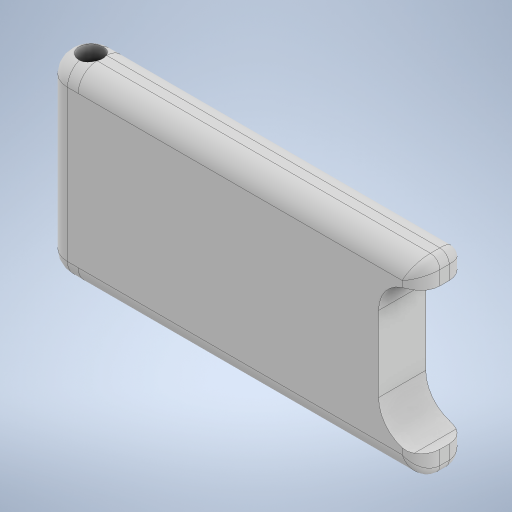
# Autodesk Inventor part: Brazo2_2
Saved by Autodesk Inventor 2024 (Build 280153000, 153)
## iProperties
Created: 2023-09-22
Part Number: Brazo2_2
Material: Genérico
Document SubType Name: Modeling
Designer: sergi
Density: 1 g/cm^3
Appearance: Valor por defecto
Author: sergi
Autodesk Inventor part; units mm, degrees
ref_plane "YZ Plane" through (0, 0, 0) normal (1, 0, 0) x (0, 1, 0)
ref_plane "XZ Plane" through (0, 0, 0) normal (0, 1, 0) x (-1, 0, 0)
ref_plane "XY Plane" through (0, 0, 0) normal (0, 0, 1) x (1, 0, 0)
sketch "Boceto1" plane through (0, 0, 0) normal (0, 0, 1) x (1, 0, 0)
  line L0 (19, -10.5) -> (-20.5, -10.5)
  arc A0 (19, -10.5) -> (20.5, -9) centre (19, -9) ccw
  line L1 (20.5, 9) -> (20.5, -9)
  arc A1 (20.5, 9) -> (19, 10.5) centre (19, 9) ccw
  line L2 (-20.5, 10.5) -> (19, 10.5)
  line L3 (-20.5, -10.5) -> (-20.5, 10.5)
  line L4 (-21, -11) -> (19, -11)
  arc A2 (19, -11) -> (21, -9) centre (19, -9) ccw
  line L5 (21, -9) -> (21, 9)
  arc A3 (21, 9) -> (19, 11) centre (19, 9) ccw
  line L6 (19, 11) -> (-21, 11)
  line L7 (-21, 11) -> (-21, -11)
  spline S0 degree 3 poles (-19.1456, -15) (-19.0838, -15) (-18.9941, -14.9843) (-18.7809, -14.9428) (-18.6401, -14.9132) (-18.3299, -14.8682) (-18.1603, -14.854) (-18, -14.854) (-17.8397, -14.854) (-17.6701, -14.8682) (-17.3599, -14.9132) (-17.2191, -14.9428) (-17.0059, -14.9843) (-16.9162, -15) (-16.8544, -15) knots 0 0 0 0 0.157027 0.157027 0.328514 0.328514 0.5 0.5 0.5 0.671486 0.671486 0.842973 0.842973 1 1 1 1
  line L8 (-16.75, -15) -> (-19.25, -15)
  line L9 (-16.75, -15) -> (-19.25, -15)
  spline S1 degree 3 poles (-19.1456, -15) (-19.0838, -15) (-18.9941, -14.9843) (-18.7809, -14.9428) (-18.6401, -14.9132) (-18.3299, -14.8682) (-18.1603, -14.854) (-18, -14.854) (-17.8397, -14.854) (-17.6701, -14.8682) (-17.3599, -14.9132) (-17.2191, -14.9428) (-17.0059, -14.9843) (-16.9162, -15) (-16.8544, -15) knots 0 0 0 0 0.157027 0.157027 0.328514 0.328514 0.5 0.5 0.5 0.671486 0.671486 0.842973 0.842973 1 1 1 1
  line L10 (-16.75, -15) -> (-19.25, -15)
  line L11 (-18, -15) -> (-18, 10.5)
  line L12 (-18, -10.5) -> (-20, -10.5)
  line L13 (-20, -10.5) -> (-20, 10.5)
  arc A4 (20, 9) -> (19, 10) centre (19, 9) ccw
  line L14 (20, 9) -> (20, -9)
  arc A5 (19, -10) -> (20, -9) centre (19, -9) ccw
  line L15 (19, -10) -> (-20, -10)
  line L16 (-20, -10) -> (-20, 10)
  line L17 (-20, 10) -> (19, 10)
  point P0 (0, 0)
  point P1 (-18, 10)
  point P2 (-20, 10)
  dimension "d0" = 0.5
  dimension "d1" = 2
  dimension "d25" = 0.5
  constraints: 22 end point, 8 point on circle, 5 point on line, 4 centre point, 2 perpendicular, 1 midpoint, 10 other
  measures "d0" distance between parallel lines of L0 L4
  measures "d1" distance of L12.start L12.end
  measures "d25" distance between parallel lines of L2 L17
extrude "Extrusión1" add sketch "Boceto1" along normal blind 5 contours L15 L13 L17 L11 | L11 L17 A4 L14 A5 L15
fillet "Empalme1" radius 2.5 2 edges at (-20, 0, 5) (-20, 0, 0)
sketch "Boceto4" plane through (0, 0, 5) normal (0, 0, 1) x (1, 0, 0)
  line L0 (-17.5, -10) -> (-17.5, 10) projected
  line L1 (18.5, 10.5) -> (19, 10.5) projected
  line L2 (18.5, 10.5) -> (18.5, -10.5) projected
  line L3 (19, -10.5) -> (18.5, -10.5) projected
  line L4 (18.5, -10.5) -> (19, -10.5) projected
  line L5 (18.5, 10.5) -> (18.5, -10.5) projected
  line L6 (19, 10.5) -> (18.5, 10.5) projected
  line L7 (20.5, 9) -> (20.5, -9)
  line L8 (25.5, -7.5) -> (19, -7.5)
  line L9 (15.5, -4) -> (15.5, 4)
  line L10 (19, 7.5) -> (25.5, 7.5)
  line L11 (25.5, 7.5) -> (25.5, -7.5)
  line L12 (25.5, -7.5) -> (15.5, 7.5) construction
  line L13 (15.5, -7.5) -> (25.5, 7.5) construction
  arc A0 (19, 7.5) -> (15.5, 4) centre (19, 4) ccw
  arc A1 (15.5, -4) -> (19, -7.5) centre (19, -4) ccw
  line L14 (-17.5, -10) -> (19, -10) projected
  arc A2 (19, -10) -> (20, -9) centre (19, -9) ccw projected
  line L15 (20, -9) -> (20, 9) projected
  arc A3 (20, 9) -> (19, 10) centre (19, 9) ccw projected
  line L16 (19, 10) -> (-17.5, 10) projected
  point P0 (0, 0)
  point P1 (20.5, 0)
  point P2 (20.5, -7.5)
  point P3 (20.5, 7.5)
  point P4 (18.5, -7.4641)
  point P5 (18.5, 7.4641)
  point P6 (20, -7.5)
  point P7 (18.5, -10)
  point P8 (20.5, 7.5)
  point P9 (20.5, -7.5)
  point P10 (18.5, 10)
  point P11 (20, 7.5)
  point P12 (20, 7.5)
  point P13 (20, -7.5)
  dimension "d15" = 10
  dimension "d16" = 15
  dimension "d17" = 3.5
  constraints: 14 end point, 4 point on circle, 4 point on line, 4 tangent, 3 midpoint, 2 centre point, 2 parallel, 1 equal radius, 1 horizontal, 1 perpendicular, 4 other
  measures "d15" distance of L12.end L10.end
  measures "d16" distance of L13.start L12.end
  measures "d17" radius of A0
extrude "Extrusión3" cut sketch "Boceto4" against normal blind 10 contours A1 L9 A0 L2 | L2 A0 L10 L15 L8 A1 | L15 L10 L7 L8 | L7 L10 L11 L8
sketch "Boceto6" plane through (19, -10, 0) normal (0, -1, 0) x (1, 0, 0)
  arc A0 (-36.5, 5) -> (-36.5, 0) centre (-36.5, 2.5) ccw projected
  point P0 (-19, 0)
  point P1 (-39, 3)
  constraints: 1 coincident
hole "Agujero2" at (-17.5, -10, 2.5) direction (0, 1, 0) diameter 2.5 end through all
fillet "Empalme3" radius 2 18 edges at (19.7071, 9.7071, 0) (0.7499, 10, 0) (-20, 10, 2.5) (-19.2678, 10, 0.7322) (-19.2678, 10, 4.2678) (0.7499, 10, 5) (19.7071, 9.7071, 5) (20, 8.25, 5) (20, -8.25, 5) (20, -8.25, 0) (20, 8.25, 0) (19.7071, -9.7071, 0) (0.7499, -10, 0) (-20, -10, 2.5) (-19.2678, -10, 0.7322) (-19.2678, -10, 4.2678) (0.7499, -10, 5) (19.7071, -9.7071, 5)
